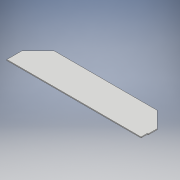
# Autodesk Inventor part: 泥除け2
Saved by Autodesk Inventor 2018 (Build 220112000, 112)
## iProperties
Created: 2017-10-09
Part Number: 泥除け2
Material: 一般
Document SubType Name: Modeling
Designer: Kosei
Density: 1 g/cm^3
Appearance: 既定
Author: Kosei
Autodesk Inventor part; units mm, degrees
ref_plane "YZ Plane" through (0, 0, 0) normal (1, 0, 0) x (0, 1, 0)
ref_plane "XZ Plane" through (0, 0, 0) normal (0, 1, 0) x (-1, 0, 0)
ref_plane "XY Plane" through (0, 0, 0) normal (0, 0, 1) x (1, 0, 0)
sketch "スケッチ1" plane through (0, 0, 0) normal (0, 0, 1) x (1, 0, 0)
  line L0 (-297.7333, 0) -> (297.7333, 0) construction
  line L1 (297.7333, 0) -> (297.7333, 0)
  line L2 (227.7333, 70) -> (-227.7333, 70)
  line L3 (-297.7333, 0) -> (-297.7333, 0)
  line L4 (0, 0) -> (0, 70) construction
  line L5 (-227.7333, 70) -> (-297.7333, 0)
  line L6 (227.7333, 70) -> (297.7333, 0)
  line L7 (-297.7333, 0) -> (297.7333, 0) construction
  line L8 (297.7333, 0) -> (297.7333, -40)
  line L9 (293.7333, -67.2) -> (-297.7333, -67.2)
  line L10 (-297.7333, -67.2) -> (-297.7333, 0)
  line L11 (-297.7333, -40) -> (297.7333, -40) construction
  line L12 (297.7333, -40) -> (293.7333, -40)
  line L13 (293.7333, -40) -> (293.7333, -67.2)
  point P0 (297.7333, 70)
  point P1 (-297.7333, 70)
  point P2 (0, 0)
  dimension "d0" = 70
  dimension "d1" = 595.4667
  dimension "d3" = 70
  dimension "d4" = 70
  dimension "d5" = 70
  dimension "d6" = 70
  dimension "d7" = 67.2
  dimension "d10" = 40
  dimension "d12" = 4
  constraints: 28 end point, 7 point on line, 5 perpendicular, 4 parallel, 2 horizontal, 2 midpoint, 1 other
  measures "d0" distance between parallel lines of L0 L2
  measures "d1" distance between parallel lines of L1 L3
  measures "d3" distance of L2.end point (-297.733, 70)
  measures "d4" distance of L3.start point (-297.733, 70)
  measures "d5" distance of L2.start point (297.733, 70)
  measures "d6" distance of L1.end point (297.733, 70)
  measures "d7" distance between parallel lines of L9 L0
  measures "d10" distance between parallel lines of L11 L0
  measures "d12" distance of L8.end L12.end
extrude "押し出し1" add sketch "スケッチ1" along normal blind 4
equation "\"d4\" = d3"
equation "\"d5\" = d3"
equation "\"d6\" = d5"
